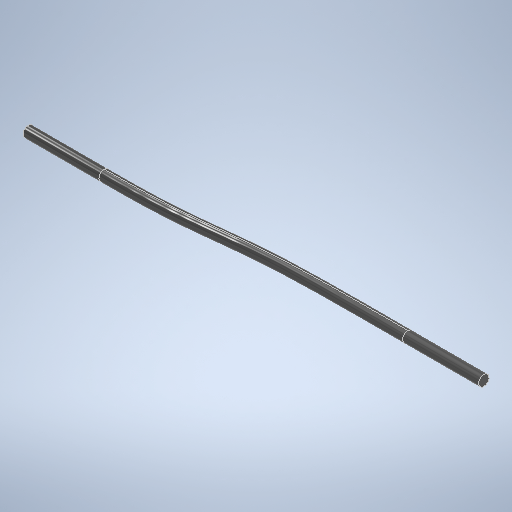
# Autodesk Inventor part: kabel2
Saved by Autodesk Inventor 2025.2 (Build 292293000, 293)
## iProperties
Created: 2024-11-20
Part Number: kabel2
Material: Generisch
Document SubType Name: Modeling
Designer: tills
Density: 1 g/cm^3
Appearance: Dunkelgrau
Author: tills
Autodesk Inventor part; units mm, degrees
ref_plane "YZ Plane" through (0, 0, 0) normal (1, 0, 0) x (0, 1, 0)
ref_plane "XZ Plane" through (0, 0, 0) normal (0, 1, 0) x (-1, 0, 0)
ref_plane "XY Plane" through (0, 0, 0) normal (0, 0, 1) x (1, 0, 0)
sketch "Skizze4" plane through (0, 0, 0) normal (0, 0, 1) x (1, 0, 0)
  line L0 (0, 0) -> (50, 0)
  line L1 (250, 8) -> (300, 8)
  spline S0 degree 4 poles (50, 0) (68.7951, 0) (100.1186, 0) (149.8812, 8.0876) (199.9698, 8) (231.2393, 8) (250, 8) knots 0 0 0 0 0 0.375049 0.625049 1 1 1 1 1
  point P0 (150, 5.9647)
  dimension "d10" = 50
  dimension "d11" = 50
  dimension "d12" = 8
  dimension "d13" = 100
  dimension "d14" = 100
  constraints: 4 end point, 4 horizontal, 3 other
  measures "d10" distance of L1.start L1.end
  measures "d11" distance of L0.start L0.end
  measures "d12" distance from line of L0.start L1
  measures "d13" horizontal distance of L0.end point (150, 5.965)
  measures "d14" horizontal distance of L1.start point (150, 5.965)
sketch "Skizze6" plane through (0, 0, 0) normal (1, 0, 0) x (0, 1, 0)
  circle A0 centre (0, 0) radius 3.5
  dimension "d15" = 7
  constraints: 1 centre point, 1 coincident
  measures "d15" diameter of A0
sweep "Sweeping2" add profiles "Skizze6" path "Skizze4" path curves L0 S0 L1
